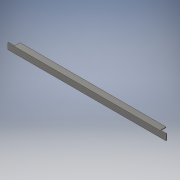
# Autodesk Inventor part: 24in1.0Lch
Saved by Autodesk Inventor 2018 (Build 220112000, 112)
## iProperties
Created: 2018-07-30
Part Number: 24in1.0Lch
Material: Steel, Mild
Document SubType Name: Modeling
Designer: Cole Tucker
Density: 7.85 g/cm^3
Appearance: Semi-Polished
Mass: 752.902 g
Surface Area: 638.49 cm^2
Volume: 95.9111 cm^3
Author: Cole Tucker
Autodesk Inventor part; units mm, degrees
ref_plane "YZ Plane" through (0, 0, 0) normal (1, 0, 0) x (0, 1, 0)
ref_plane "XZ Plane" through (0, 0, 0) normal (0, 1, 0) x (-1, 0, 0)
ref_plane "XY Plane" through (0, 0, 0) normal (0, 0, 1) x (1, 0, 0)
sketch "Sketch1" plane through (0, 0, 0) normal (1, 0, 0) x (0, 1, 0)
  line L0 (0, 0) -> (25.4, 0)
  line L1 (25.4, 0) -> (25.4, -25.4)
  line L2 (25.4, -25.4) -> (23.8252, -25.4)
  line L3 (0, -1.5748) -> (0, 0)
  line L4 (25.4, 0) -> (22.225, 0) construction
  line L5 (22.225, 0) -> (22.225, -3.175) construction
  line L6 (22.225, -3.175) -> (25.4, -3.175) construction
  line L7 (25.4, -3.175) -> (25.4, 0) construction
  line L8 (25.4, -25.4) -> (22.225, -25.4) construction
  line L9 (0, 0) -> (0, -3.175) construction
  line L10 (1.6002, -3.175) -> (20.6248, -3.175)
  line L11 (22.225, -23.7998) -> (22.225, -4.7752)
  arc A0 (22.225, -23.7998) -> (23.8252, -25.4) centre (23.8252, -23.7998) ccw
  arc A1 (0, -1.5748) -> (1.6002, -3.175) centre (1.6002, -1.5748) ccw
  arc A2 (22.225, -4.7752) -> (20.6248, -3.175) centre (20.6248, -4.7752) ccw
  point P0 (0, -25.4)
  dimension "d0" = 25.4
  dimension "d1" = 25.4
  dimension "d2" = 3.175
  dimension "d3" = 3.175
  dimension "d4" = 3.175
  dimension "d5" = 3.175
  dimension "d6" = 1.6002
  dimension "d7" = 1.6002
  constraints: 24 end point, 8 point on line, 6 point on circle, 6 tangent, 4 parallel, 3 centre point, 2 horizontal, 2 perpendicular, 1 equal radius
  measures "d0" distance of L1.end point (0, -25.4)
  measures "d1" distance of L0.end L1.end
  measures "d2" distance of L6.end L5.end
  measures "d3" distance of L5.end L4.end
  measures "d4" distance of L1.end L8.end
  measures "d5" distance of L0.start L9.end
  measures "d6" radius of A0
  measures "d7" radius of A1
extrude "Extrusion1" add sketch "Sketch1" along normal blind 660.4
sketch "Sketch2" plane through (0, 25.4, 0) normal (0, 1, 0) x (1, 0, 0)
  line L0 (0, 25.4) -> (0, 23.7998) projected
  line L1 (0, 3.175) -> (660.4, 3.175) projected
  line L2 (0, 25.4) -> (25.4, 25.4)
  line L3 (25.4, 25.4) -> (25.4, 3.175)
  line L4 (25.4, 3.175) -> (0, 3.175)
  line L5 (0, 3.175) -> (0, 25.4)
  line L6 (660.4, 25.4) -> (635, 25.4)
  line L7 (635, 25.4) -> (635, 3.175)
  line L8 (635, 3.175) -> (660.4, 3.175)
  line L9 (660.4, 3.175) -> (660.4, 25.4)
  point P0 (0, 0)
  dimension "d10" = 25.4
  dimension "d11" = 25.4
  dimension "d12" = 22.225
  constraints: 16 end point, 4 parallel, 2 horizontal, 2 perpendicular, 1 point on line
  measures "d10" distance of L3.end L4.end
  measures "d11" distance of L8.end L7.end
  measures "d12" distance of L6.end L7.end
extrude "Extrusion2" cut sketch "Sketch2" against normal blind 25.4
body "Solid1"
